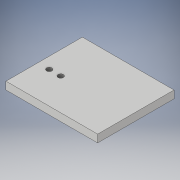
# Autodesk Inventor part: Load cell support
Saved by Autodesk Inventor 2019 (Build 230136000, 136)
## iProperties
Created: 2021-03-05
Part Number: Load cell support
Material: Generic
Document SubType Name: Modeling
Designer: User
Density: 1 g/cm^3
Appearance: Default
Author: User
Autodesk Inventor part; units mm, degrees
ref_plane "YZ Plane" through (0, 0, 0) normal (1, 0, 0) x (0, 1, 0)
ref_plane "XZ Plane" through (0, 0, 0) normal (0, 1, 0) x (-1, 0, 0)
ref_plane "XY Plane" through (0, 0, 0) normal (0, 0, 1) x (1, 0, 0)
sketch "Sketch1" plane through (0, 0, 0) normal (0, 1, 0) x (-1, 0, 0)
  line L0 (70, 41.6667) -> (-50, 41.6667)
  line L1 (-50, 41.6667) -> (-50, -58.3333)
  line L2 (-50, -58.3333) -> (70, -58.3333)
  line L3 (70, -58.3333) -> (70, 41.6667)
  point P0 (0, 0)
  dimension "d0" = 100
  dimension "d1" = 120
  dimension "d2" = 70
  dimension "d3" = 41.6667
  constraints: 8 end point, 2 parallel, 1 horizontal, 1 perpendicular
  measures "d0" distance between parallel lines of L2 L0
  measures "d1" distance between parallel lines of L1 L3
  measures "d2" distance from line of point (0, 0) L3
  measures "d3" distance from line of point (0, 0) L0
extrude "Extrusion1" add sketch "Sketch1" along normal blind 10
sketch "Sketch2" plane through (0, 10, 0) normal (0, 1, 0) x (1, 0, 0)
  circle A0 centre (-40, 0) radius 3.5
  circle A1 centre (-55, 0) radius 3.5
  line L0 (-70, 58.3333) -> (-70, -41.6667) projected
  point P0 (0, 0)
  dimension "d6" = 7
  dimension "d7" = 7
  dimension "d8" = 30
  dimension "d9" = 15
  dimension "d12" = 15
  dimension "d13" = 40
  constraints: 2 centre point
  measures "d6" diameter of A0
  measures "d7" diameter of A1
  measures "d8" distance from line of A0.centre L0
  measures "d9" distance of A0.centre A1.centre
  measures "d12" distance from line of A1.centre L0
  measures "d13" distance of point (0, 0) A0.centre
extrude "Extrusion2" cut sketch "Sketch2" against normal blind 5
thread "Thread1" size "M7x1" class "6H" standard "ANSI Metric M Profile" full length
thread "Thread2" size "M7x1" class "6H" standard "ANSI Metric M Profile" full length
body "Solid1"
